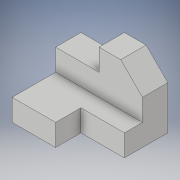
# Autodesk Inventor part: 410571040練習一
Saved by Autodesk Inventor 2017 (Build 210142000, 142)
## iProperties
Part Number: 410571040練習一
Material: 一般
Document SubType Name: Modeling
Designer: user
Density: 1 g/cm^3
Appearance: 預設
Author: user
Autodesk Inventor part; units mm, degrees
ref_plane "YZ Plane" through (0, 0, 0) normal (1, 0, 0) x (0, 1, 0)
ref_plane "XZ Plane" through (0, 0, 0) normal (0, 1, 0) x (-1, 0, 0)
ref_plane "XY Plane" through (0, 0, 0) normal (0, 0, 1) x (1, 0, 0)
sketch "草圖1" plane through (0, 0, 0) normal (0, 1, 0) x (-1, 0, 0)
  line L0 (0, 0) -> (-24, 0)
  line L1 (-24, 0) -> (-24, -14)
  line L2 (-24, -14) -> (-48, -14)
  line L3 (-48, -14) -> (-48, -38)
  line L4 (-48, -38) -> (0, -38)
  line L5 (0, -38) -> (0, 0)
  dimension "d0" = 24
  dimension "d1" = 14
  dimension "d2" = 38
  dimension "d3" = 48
  constraints: 12 end point, 5 perpendicular, 1 horizontal
  measures "d0" distance of L0.start L0.end
  measures "d1" distance of L0.end L1.end
  measures "d2" distance of L4.end L0.start
  measures "d3" distance of L3.end L4.end
extrude "擠出1" add sketch "草圖1" along normal blind 12
sketch "草圖2" plane through (48, 0, -38) normal (0, 0, -1) x (-1, 0, 0)
  line L0 (48, 12) -> (24, 12) projected
  line L1 (48, 12) -> (48, 24)
  line L2 (48, 24) -> (24, 24)
  line L3 (24, 24) -> (24, 36)
  line L4 (24, 36) -> (12, 36)
  line L5 (12, 36) -> (0, 24)
  line L6 (24, 12) -> (0, 12) projected
  line L7 (0, 24) -> (0, 12)
  line L8 (0, 12) -> (48, 12)
  point P0 (48, 0)
  dimension "d6" = 12
  dimension "d7" = 24
  dimension "d8" = 12
  dimension "d9" = 12
  constraints: 14 end point, 3 perpendicular, 2 parallel, 1 point on line, 1 vertical
  measures "d6" distance of L0.start L1.end
  measures "d7" distance of L1.end L2.end
  measures "d8" horizontal distance of L5.end L4.end
  measures "d9" horizontal distance of L5.end L4.end
extrude "擠出2" add sketch "草圖2" against normal blind 14
